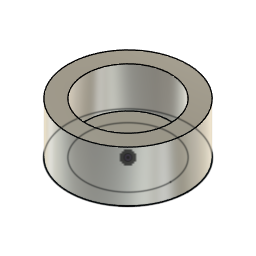
l01_first_print (Autodesk Fusion 360 design; units mm, degrees)
part number: 2025-08-20-18-05-59-878
Autodesk Fusion 360 part; units mm, degrees
sketch "Sketch1" plane through (0, 0, 0) normal (0, 0, 1) x (1, 0, 0)
sketch "Sketch2" plane through (0, 0, 0) normal (0, 0, 1) x (1, 0, 0)
  circle A0 centre (0, 0) radius 12.5
  circle A1 centre (0, 0) radius 17.5
  dimension "d2" = 25
  dimension "d3" = 35
  constraint coincident A0.centre A1.centre
  measures "d2" diameter of A0
  measures "d3" diameter of A1
extrude "Extrude1" add sketch "Sketch2" along normal blind 13 contours A0
extrude "Extrude2" cut 1 faces at (-3.3879, -0.621, 13) along direction (0, 0, -1) blind 13
extrude "Extrude3" add sketch "Sketch2" along normal blind 7
extrude "Extrude4" add sketch "Sketch2" along normal blind 17 contours A0
extrude "Extrude5" cut 1 faces at (-3.3879, -0.621, 17) along direction (0, 0, -1) blind 15
extrude "Extrude6" cut 1 faces at (15.7682, -0.8694, 7) along direction (0, 0, -1) blind 7
extrude "Extrude7" cut 1 faces at (-3.3879, -0.621, 2) along direction (0, 0, -1) blind 2
extrude "Extrude8" add sketch "Sketch2" along normal blind 10
extrude "Extrude9" add sketch "Sketch2" along normal blind 3 contours A0
extrude "Extrude10" cut 1 faces at (15.7682, -0.8694, 10) along direction (0, 0, -1) blind 10
extrude "Extrude11" add sketch "Sketch2" along normal blind 15
